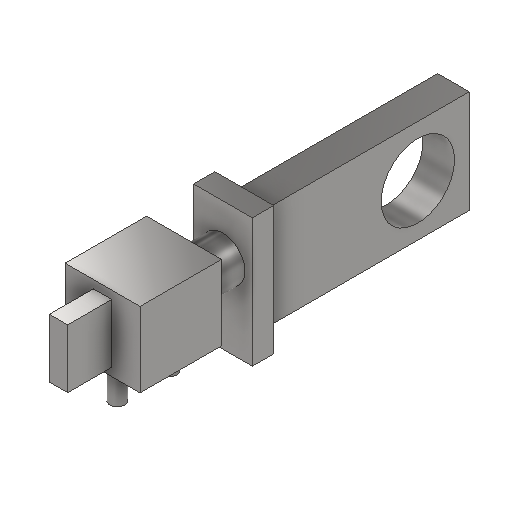
# Autodesk Inventor part: gate_valve
Saved by Autodesk Inventor 2026.2 (Build 302298000, 298)
## iProperties
Created: 2026-03-12
Part Number: gate_valve
Material: ステンレス鋼 440C
Document SubType Name: Modeling
Designer: zetsu
Density: 7.75 g/cm^3
Appearance: 半つや出し
Author: zetsu
Autodesk Inventor part; units mm, degrees
ref_plane "YZ Plane" through (0, 0, 0) normal (1, 0, 0) x (0, 1, 0)
ref_plane "XZ Plane" through (0, 0, 0) normal (0, 1, 0) x (-1, 0, 0)
ref_plane "XY Plane" through (0, 0, 0) normal (0, 0, 1) x (1, 0, 0)
sketch "スケッチ1" plane through (0, 0, 0) normal (0, 0, 1) x (1, 0, 0)
  line L0 (-21.5, 70) -> (21.5, 70)
  line L1 (21.5, 70) -> (21.5, -70)
  line L2 (21.5, -70) -> (-21.5, -70)
  line L3 (-21.5, -70) -> (-21.5, 70)
  line L4 (0, 0) -> (0, 119.7225) construction
  line L5 (0, 0) -> (105.4922, 0) construction
  dimension "d0" = 43
  dimension "d1" = 140
  constraints: 12 end point, 2 horizontal, 2 parallel, 1 perpendicular, 1 vertical, 2 other
  measures "d0" distance of L0.end L0.start
  measures "d1" distance of L1.end L0.end
extrude "押し出し1" add sketch "スケッチ1" along normal blind 285
sketch "スケッチ2" plane through (0, 0, 285) normal (0, 0, 1) x (1, 0, 0)
  point P0 (0, 0)
sketch "スケッチ3" plane through (0, 0, 285) normal (0, 0, 1) x (1, 0, 0)
  line L0 (-40, 87.5) -> (40, 87.5)
  line L1 (40, 87.5) -> (40, -87.5)
  line L2 (40, -87.5) -> (-40, -87.5)
  line L3 (-40, -87.5) -> (-40, 87.5)
  line L4 (0, 0) -> (0, 125.4617) construction
  line L5 (0, 0) -> (95.6188, 0) construction
  dimension "d4" = 80
  dimension "d5" = 175
  constraints: 12 end point, 2 horizontal, 2 parallel, 1 perpendicular, 1 vertical, 2 other
  measures "d4" distance of L0.end L0.start
  measures "d5" distance of L1.end L0.end
extrude "押し出し2" add sketch "スケッチ3" along normal blind 29
sketch "スケッチ4" plane through (0, 0, 314) normal (0, 0, 1) x (1, 0, 0)
  circle A0 centre (0, 19.5) radius 30
  line L0 (40, 87.5) -> (-40, 87.5) projected
  point P0 (0, 0)
  point P1 (0, 87.5)
  dimension "d8" = 60
  dimension "d9" = 68
  constraints: 1 centre point, 1 midpoint
  measures "d8" diameter of A0
  measures "d9" distance of A0.centre point (0, 87.5)
extrude "押し出し3" add sketch "スケッチ4" along normal blind 53
sketch "スケッチ5" plane through (0, 19.5, 367) normal (0, 0, 1) x (1, 0, 0)
  line L0 (-51, 51) -> (51, 51)
  line L1 (51, 51) -> (51, -51)
  line L2 (51, -51) -> (-51, -51)
  line L3 (-51, -51) -> (-51, 51)
  line L4 (0, 0) -> (0, 75.1784) construction
  line L5 (0, 0) -> (69.351, 0) construction
  point P0 (0, -19.5)
  dimension "d12" = 102
  dimension "d13" = 102
  constraints: 12 end point, 2 horizontal, 2 parallel, 1 perpendicular, 1 vertical, 2 other
  measures "d12" distance of L0.end L0.start
  measures "d13" distance of L1.end L0.end
extrude "押し出し4" add sketch "スケッチ5" along normal blind 111
sketch "スケッチ6" plane through (0, 19.5, 478) normal (0, 0, 1) x (1, 0, 0)
  line L0 (-12.5, 40) -> (12.5, 40)
  line L1 (12.5, 40) -> (12.5, -40)
  line L2 (12.5, -40) -> (-12.5, -40)
  line L3 (-12.5, -40) -> (-12.5, 40)
  line L4 (0, 0) -> (0, 47.6944) construction
  line L5 (0, 0) -> (61.4102, 0) construction
  point P0 (0, -19.5)
  dimension "d16" = 25
  dimension "d17" = 80
  constraints: 12 end point, 2 horizontal, 2 parallel, 1 perpendicular, 1 vertical, 2 other
  measures "d16" distance of L0.end L0.start
  measures "d17" distance of L1.end L0.end
extrude "押し出し5" add sketch "スケッチ6" along normal blind 60
sketch "スケッチ7" plane through (-51, -31.5, 367) normal (0, -1, 0) x (1, 0, 0)
  circle A0 centre (51, 91) radius 10
  circle A1 centre (51, 20) radius 10
  line L0 (0, 111) -> (102, 111) projected
  line L1 (0, 0) -> (102, 0) projected
  point P0 (51, -367)
  point P1 (51, 111)
  point P2 (51, 0)
  dimension "d20" = 20
  dimension "d21" = 20
  dimension "d22" = 20
  dimension "d23" = 20
  constraints: 2 centre point, 2 midpoint
  measures "d20" diameter of A0
  measures "d21" diameter of A1
  measures "d22" distance of A0.centre point (51, 111)
  measures "d23" distance of point (51, 0) A1.centre
extrude "押し出し6" add sketch "スケッチ7" along normal blind 45
sketch "スケッチ8" plane through (-21.5, -70, 0) normal (-1, 0, 0) x (0, 0, 1)
  circle A0 centre (70, 70) radius 50
  line L0 (0, 140) -> (0, 0) projected
  point P0 (0, 70)
  point P1 (0, 70)
  dimension "d26" = 100
  dimension "d27" = 70
  constraints: 1 centre point, 1 midpoint
  measures "d26" diameter of A0
  measures "d27" distance of point (0, 70) A0.centre
extrude "押し出し7" cut sketch "スケッチ8" against normal through all
